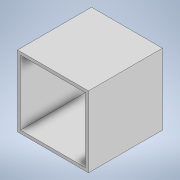
# Autodesk Inventor part: body
Saved by Autodesk Inventor 2022.2 (Build 262287030, 287C)
## iProperties
Created: 2022-02-20
Part Number: body
Material: Generic
Document SubType Name: Modeling
Designer: Nakai
Density: 1 g/cm^3
Appearance: Default
Author: Nakai
Autodesk Inventor part; units mm, degrees
ref_plane "YZ Plane" through (0, 0, 0) normal (1, 0, 0) x (0, 1, 0)
ref_plane "XZ Plane" through (0, 0, 0) normal (0, 1, 0) x (-1, 0, 0)
ref_plane "XY Plane" through (0, 0, 0) normal (0, 0, 1) x (1, 0, 0)
sketch "Sketch1" plane through (0, 0, 0) normal (0, 0, 1) x (1, 0, 0)
  line L0 (0, 0) -> (70, 0)
  line L1 (70, 0) -> (70, 70)
  line L2 (70, 70) -> (0, 70)
  line L3 (0, 70) -> (0, 0)
  dimension "d0" = 70
  dimension "d1" = 70
  constraints: 8 end point, 2 parallel, 1 horizontal, 1 perpendicular
  measures "d0" distance of L2.end L1.end
  measures "d1" distance of L1.end L0.end
extrude "Extrusion1" add sketch "Sketch1" along normal blind 3
sketch "Sketch2" plane through (0, 0, 3) normal (0, 0, 1) x (1, 0, 0)
  line L0 (70, 70) -> (0, 70) projected
  line L1 (70, 0) -> (70, 70) projected
  line L2 (0, 70) -> (70, 70)
  line L3 (70, 70) -> (70, 0)
  line L4 (70, 0) -> (0, 0)
  line L5 (0, 0) -> (0, 70)
  line L6 (3, 67) -> (67, 67)
  line L7 (67, 67) -> (67, 3)
  line L8 (67, 3) -> (3, 3)
  line L9 (3, 3) -> (3, 67)
  dimension "d4" = 3
  constraints: 16 end point, 4 parallel, 2 perpendicular, 1 horizontal, 3 other
  measures "d4" distance between parallel lines of L5 L9
extrude "Extrusion2" add sketch "Sketch2" along normal blind 70
body "Solid1"
